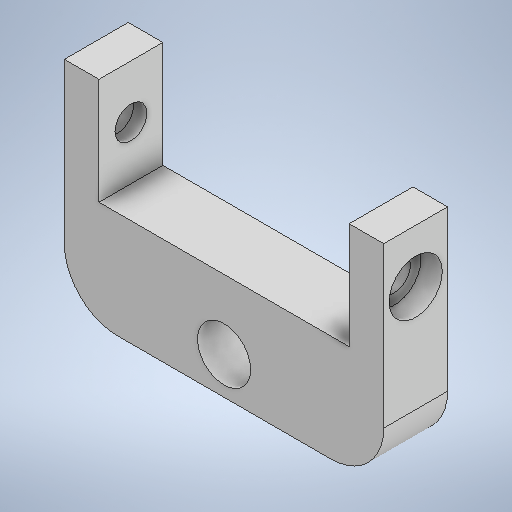
# Autodesk Inventor part: partContainerConnector
Saved by Autodesk Inventor 2025.3 (Build 293356000, 356)
## iProperties
Created: 2025-04-28
Part Number: partContainerConnector
Material: 일반
Document SubType Name: Modeling
Designer: SEON
Density: 1 g/cm^3
Appearance: 기본값
Author: SEON
Autodesk Inventor part; units mm, degrees
ref_plane "YZ Plane" through (0, 0, 0) normal (1, 0, 0) x (0, 1, 0)
ref_plane "XZ Plane" through (0, 0, 0) normal (0, 1, 0) x (-1, 0, 0)
sketch "스케치1" plane through (0, 0, 0) normal (0, 0, 1) x (1, 0, 0)
  line L0 (0, 0) -> (0, 20)
  line L1 (0, 20) -> (3.25, 20)
  line L2 (3.25, 20) -> (3.25, 10)
  line L3 (3.25, 10) -> (26.75, 10)
  line L4 (26.75, 10) -> (26.75, 20)
  line L5 (26.75, 20) -> (30, 20)
  line L6 (30, 20) -> (30, 0)
  line L7 (30, 0) -> (0, 0)
  circle A0 centre (15, 3.5) radius 2.5
  point P0 (15, 10)
  point P1 (15, 0)
  dimension "d0" = 23.5
  dimension "d1" = 10
  dimension "d2" = 30
  dimension "d6" = 10
  dimension "d14" = 5
  dimension "d17" = 3.5
  constraints: 16 end point, 6 perpendicular, 2 midpoint, 2 point on line, 2 vertical alignment, 1 centre point, 1 vertical
  measures "d0" distance between parallel lines of L4 L2
  measures "d1" distance between parallel lines of L7 L3
  measures "d2" distance between parallel lines of L0 L6
  measures "d6" distance between parallel lines of L3 L1
  measures "d14" diameter of A0
  measures "d17" distance from line of L7 A0.centre
extrude "돌출1" add sketch "스케치1" along normal blind 6
sketch "스케치2" plane through (30, 0, 0) normal (1, 0, 0) x (0, 0, -1)
  line L0 (-6, 20) -> (-6, 10) projected
  line L1 (0, 20) -> (-6, 20) projected
  point P0 (0, 0)
  point P1 (-3, 15)
  point P2 (-6, 15)
  point P3 (-3, 20)
  constraints: 2 midpoint, 1 horizontal alignment, 1 vertical alignment
hole "구멍1" at (30, 15, 3) direction (-1, 0, 0) diameter 3 end through all counterbore diameter 5 counterbore depth 2
ref_plane "작업 평면1" through (15, 0, 0) normal (1, 0, 0) x (0, 0, -1)
mirror "미러1" about plane through (15, 0, 0) normal (1, 0, 0) of "구멍1"
fillet "모깎기1" radius 5 2 edges at (30, 0, 3) (0, 0, 3)
